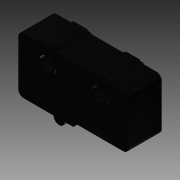
# Autodesk Inventor part: Pololu #1402 Snap-Action Switch
Saved by Autodesk Inventor 2014 SP1 (Build 180222100, 222)
## iProperties
Created: 2013-12-20
Part Number: Pololu #1402 Snap-Action Switch
Material: PC/ABS Plastic
Document SubType Name: Modeling
Designer: JustinIndra
Density: 0.357273 g/cm^3
Appearance: Smooth - Black
Author: JustinIndra
Autodesk Inventor part; units mm, degrees
ref_plane "YZ Plane" through (0, 0, 0) normal (1, 0, 0) x (0, 1, 0)
ref_plane "XZ Plane" through (0, 0, 0) normal (0, 1, 0) x (-1, 0, 0)
ref_plane "XY Plane" through (0, 0, 0) normal (0, 0, 1) x (1, 0, 0)
sketch "Sketch1" plane through (0, 0, 0) normal (0, 1, 0) x (-1, 0, 0)
  line L0 (10, -5.1) -> (-10, -5.1)
  line L1 (-10, -5.1) -> (-10, 5.1)
  line L2 (-10, 5.1) -> (10, 5.1)
  line L3 (10, 5.1) -> (10, -5.1)
  line L4 (6.45, 5.1) -> (5.95, 5.5)
  line L5 (5.95, 5.5) -> (3.55, 5.5)
  line L6 (3.55, 5.5) -> (3.05, 5.1)
  line L7 (-3.05, 5.1) -> (-3.55, 5.5)
  line L8 (-3.55, 5.5) -> (-5.95, 5.5)
  line L9 (-5.95, 5.5) -> (-6.45, 5.1)
  point P0 (0, 0)
  point P1 (0, -5.1)
  point P2 (10, 0)
  point P3 (4.75, 5.5)
  point P4 (-4.75, 5.5)
  dimension "d0" = 20
  dimension "d1" = 10.2
  dimension "d2" = 0.4
  dimension "d3" = 0.5
  dimension "d4" = 2.4
  dimension "d5" = 5.25
  dimension "d6" = 9.5
  constraints: 20 end point, 7 equal length, 4 midpoint, 4 point on line, 2 perpendicular, 1 collinear, 1 horizontal, 1 horizontal alignment, 1 vertical alignment
  measures "d0" distance of L1.end L2.end
  measures "d1" distance of L0.end L1.end
  measures "d2" distance between parallel lines of L2 L5
  measures "d3" horizontal distance of L4.end L4.start
  measures "d4" distance of L4.end L5.end
  measures "d5" distance from line of L3 point (4.75, 5.5)
  measures "d6" distance of point (4.75, 5.5) point (-4.75, 5.5)
extrude "Extrusion1" add sketch "Sketch1" along normal mid plane 6
sketch "Sketch2" plane through (0, 3, 0) normal (0, 1, 0) x (1, 0, 0)
  line L0 (10, -5.1) -> (10, 5.1) projected
  line L1 (10, 5.1) -> (-10, 5.1) projected
  line L2 (-10, 5.1) -> (-10, -5.1) projected
  line L3 (0, 5.1) -> (0.5, 4.4)
  line L4 (0.5, 4.4) -> (10, 4.4)
  point P0 (0, 0)
  dimension "d9" = 10.5
  dimension "d10" = 0.5
  dimension "d11" = 0.7
  constraints: 4 end point, 1 midpoint, 1 perpendicular, 1 point on line
  measures "d9" distance from line of L2 L3.end
  measures "d10" horizontal distance of L3.start L3.end
  measures "d11" distance between parallel lines of L4 L1
extrude "Extrusion2" cut sketch "Sketch2" against normal through all
sketch "Sketch4" plane through (0, 3, 0) normal (0, 1, 0) x (1, 0, 0)
  circle A0 centre (-4.75, -2.6) radius 1.7
  circle A1 centre (4.75, -2.6) radius 1.7
  line L0 (-6.45, -2.6) -> (-3.05, -2.6)
  line L1 (-3.05, -2.6) -> (-3.05, -5.1)
  line L2 (-3.05, -5.1) -> (-6.45, -5.1)
  line L3 (-6.45, -5.1) -> (-6.45, -2.6)
  line L4 (3.05, -2.6) -> (6.45, -2.6)
  line L5 (6.45, -2.6) -> (6.45, -5.1)
  line L6 (6.45, -5.1) -> (3.05, -5.1)
  line L7 (3.05, -5.1) -> (3.05, -2.6)
  line L8 (-10, -5.1) -> (-6.45, -5.1) projected
  point P0 (0, 0)
  dimension "d18" = 3.4
  dimension "d21" = 2.5
  constraints: 16 end point, 4 horizontal alignment, 4 parallel, 2 coincident, 2 horizontal, 2 perpendicular, 1 collinear, 4 other
  measures "d21" distance from line of L8 point (-4.75, -2.6)
extrude "Extrusion4" add sketch "Sketch4" along normal blind 0.2
mirror "Mirror1" about plane through (0, 0, 0) normal (0, 1, 0) of "Extrusion4"
sketch "Sketch5" plane through (0, 3.2, 0) normal (0, 1, 0) x (1, 0, 0)
  arc A0 (-3.05, -2.6) -> (-6.45, -2.6) centre (-4.75, -2.6) ccw projected
  circle A1 centre (-4.75, -2.6) radius 1.2
  circle A2 centre (4.75, -2.6) radius 1.2
  line L0 (3.05, -5.1) -> (6.45, -5.1) projected
  point P0 (0, 0)
  point P1 (4.75, -5.1)
  dimension "d22" = 2.4
  constraints: 2 centre point, 1 coincident, 1 equal radius, 1 horizontal alignment, 1 midpoint, 1 vertical alignment
  measures "d22" diameter of A1
extrude "Extrusion5" cut sketch "Sketch5" against normal through all
sketch "Sketch6" plane through (0, 0, 0) normal (0, 1, 0) x (-1, 0, 0)
  line L0 (2.6, -5.1) -> (4.6, -5.1)
  line L1 (4.6, -5.1) -> (4.6, -6.1)
  line L2 (4.6, -6.1) -> (2.6, -6.1)
  line L3 (2.6, -6.1) -> (2.6, -5.1)
  line L4 (0, -5.1) -> (10, -5.1) projected
  line L5 (10, -5.1) -> (10, 5.1) projected
  circle A0 centre (3.6, -6.1) radius 1
  point P0 (0, 0)
  dimension "d25" = 6.4
  dimension "d26" = 2
  dimension "d27" = 1
  constraints: 8 end point, 2 parallel, 1 coincident, 1 collinear, 1 horizontal, 1 horizontal alignment, 1 midpoint, 1 perpendicular, 2 other
  measures "d25" distance from line of L5 point (3.6, -6.1)
  measures "d26" distance between parallel lines of L3 L1
  measures "d27" distance between parallel lines of L0 L2
extrude "Extrusion6" add sketch "Sketch6" along normal mid plane 4
fillet "Fillet1" radius 1 4 edges at (-10, 0, -5.1) (10, 0, -4.4) (10, 0, 5.1) (-10, 0, 5.1)
body "Solid1"
